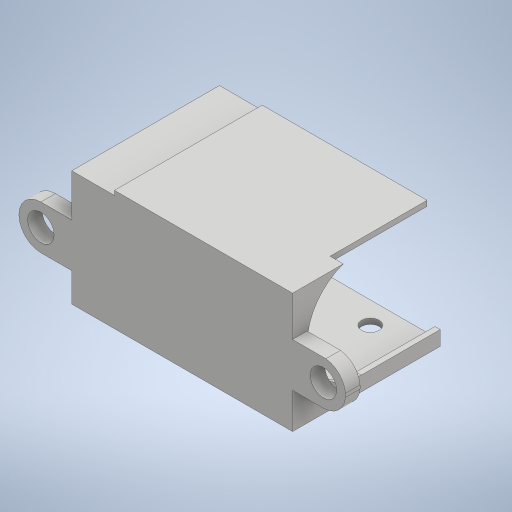
# Autodesk Inventor part: MotorMount
Saved by Autodesk Inventor 2023 (Build 270158000, 158)
## iProperties
Created: 2019-11-11
Part Number: MotorMount
Material: Generic
Document SubType Name: Modeling
Designer: neera
Density: 1 g/cm^3
Appearance: Default
Author: neera
Autodesk Inventor part; units mm, degrees
ref_plane "YZ Plane" through (0, 0, 0) normal (1, 0, 0) x (0, 1, 0)
ref_plane "XZ Plane" through (0, 0, 0) normal (0, 1, 0) x (-1, 0, 0)
ref_plane "XY Plane" through (0, 0, 0) normal (0, 0, 1) x (1, 0, 0)
sketch "Sketch1" plane through (0, 0, 0) normal (0, 1, 0) x (-1, 0, 0)
  line L0 (17.1623, 10.1297) -> (-30.5377, 10.1297)
  line L1 (-30.5377, 34.9297) -> (7.4623, 34.9297)
  line L2 (7.4623, 34.9297) -> (7.4623, 33.9297)
  line L3 (7.4623, 33.9297) -> (17.1623, 33.9297)
  line L4 (17.1623, 33.9297) -> (17.1623, 10.1297)
  line L5 (-31.7377, 8.9297) -> (18.3623, 8.9297)
  line L6 (18.3623, 8.9297) -> (18.3623, 35.1297)
  line L7 (18.3623, 35.1297) -> (8.6623, 35.1297)
  line L8 (8.6623, 35.1297) -> (8.6623, 36.1297)
  line L9 (8.6623, 36.1297) -> (-31.7377, 36.1297)
  line L10 (-30.5377, 10.1297) -> (-30.5377, 34.9297)
  line L11 (-31.7377, 8.9297) -> (-31.7377, 36.1297)
  point P0 (0, 0)
  dimension "d0" = 47.7
  dimension "d1" = 23.8
  dimension "d2" = 9.7
  dimension "d3" = 1
  dimension "d4" = 1.2
  dimension "d5" = 1.2
  dimension "d6" = 1.2
  dimension "d7" = 1.2
  dimension "d8" = 1.2
  dimension "d19" = 1.2
  constraints: 24 end point, 8 perpendicular, 2 horizontal
  measures "d0" distance of L0.start L0.end
  measures "d1" distance of L3.end L0.start
  measures "d2" distance of L2.end L3.end
  measures "d3" distance of L1.end L2.end
  measures "d4" distance between parallel lines of L0 L5
  measures "d5" distance between parallel lines of L6 L4
  measures "d6" distance between parallel lines of L3 L7
  measures "d7" distance between parallel lines of L2 L8
  measures "d8" distance between parallel lines of L1 L9
  measures "d19" distance between parallel lines of L10 L11
extrude "Extrusion3" add sketch "Sketch1" along normal blind 33.5
sketch "Sketch3" plane through (0, 0, 0) normal (0, -1, 0) x (1, 0, 0)
  line L0 (30.5377, 34.9297) -> (-7.4623, 34.9297) projected
  line L1 (30.5377, 34.9297) -> (30.5377, 10.1297) projected
  line L2 (30.5377, 34.9297) -> (30.5377, 10.1297)
  line L3 (-17.1623, 10.1297) -> (30.5377, 10.1297) projected
  line L4 (30.5377, 10.1297) -> (-17.1623, 10.1297)
  line L5 (-17.1623, 33.9297) -> (-17.1623, 10.1297) projected
  line L6 (-17.1623, 10.1297) -> (-17.1623, 33.9297)
  line L7 (-7.4623, 33.9297) -> (-7.4623, 34.9297) projected
  line L8 (-17.1623, 33.9297) -> (-7.4623, 33.9297)
  line L9 (-7.4623, 33.9297) -> (-7.4623, 34.9297)
  line L10 (-7.4623, 34.9297) -> (30.5377, 34.9297)
  point P0 (0, 0)
  constraints: 12 end point, 4 perpendicular, 2 collinear
extrude "Extrusion4" add sketch "Sketch3" against normal blind 1.2
sketch "Sketch4" plane through (31.7377, 0, 8.9297) normal (0, 0, -1) x (-1, 0, 0)
  arc A0 (29.9, 16.8) -> (38.3, 16.8) centre (34.1, 16.8) ccw
  line L0 (50.1, 0) -> (50.1, 33.5) projected
  line L1 (0, 0) -> (50.1, 0) projected
  line L2 (29.9, 16.8) -> (29.9, 33.5)
  line L3 (29.9, 33.5) -> (38.3, 33.5)
  line L4 (0, 33.5) -> (50.1, 33.5) projected
  line L5 (38.3, 33.5) -> (38.3, 16.8)
  circle A1 centre (43.65, 28.5) radius 2
  circle A2 centre (43.65, 8.5) radius 2
  circle A3 centre (10.85, 8.5) radius 2
  circle A4 centre (10.85, 28.5) radius 2
  point P0 (31.7377, 0)
  dimension "d24" = 16
  dimension "d25" = 16.8
  dimension "d26" = 4.2
  dimension "d27" = 4
  dimension "d28" = 6.45
  dimension "d29" = 5
  dimension "d30" = 4
  dimension "d31" = 6.45
  dimension "d32" = 20
  dimension "d33" = 4
  dimension "d34" = 4
  dimension "d35" = 32.8
  dimension "d36" = 20
  dimension "d37" = 5
  dimension "d38" = 0
  constraints: 6 end point, 5 centre point, 2 point on circle, 2 tangent, 2 vertical, 1 point on line
  measures "d24" distance from line of L0 A0.centre
  measures "d25" distance from line of L1 A0.centre
  measures "d26" radius of A0
  measures "d27" diameter of A1
  measures "d28" distance from line of L0 A1.centre
  measures "d29" distance from line of L4 A1.centre
  measures "d30" diameter of A2
  measures "d31" distance from line of L0 A2.centre
  measures "d32" distance of A1.centre A2.centre
  measures "d33" diameter of A3
  measures "d34" diameter of A4
  measures "d35" distance of A2.centre A3.centre
  measures "d36" distance of A3.centre A4.centre
  measures "d37" distance from line of A4.centre L4
  measures "d38" horizontal distance of A3.centre A4.centre
extrude "Extrusion5" cut sketch "Sketch4" against normal blind 5
sketch "Sketch5" plane through (31.7377, 0, 36.1297) normal (1, 0, 0) x (0, 0, -1)
  arc A0 (-0.7, 15.6) -> (23.9, 15.6) centre (11.6, 15.6) ccw
  line L0 (0, 0) -> (27.2, 0) projected
  line L1 (27.2, 0) -> (27.2, 33.5) projected
  line L2 (23.9, 15.6) -> (23.9, 33.5)
  line L3 (27.2, 33.5) -> (1, 33.5) projected
  line L4 (1, 33.5) -> (0, 33.5) projected
  line L5 (-0.7, 15.6) -> (18, 15.6) construction
  line L6 (0.1, 33.5) -> (23.9, 33.5)
  line L7 (-0.7, 15.6) -> (0, 15.6)
  line L8 (0, 0) -> (0, 33.5) projected
  line L9 (0, 15.6) -> (0, 33.5)
  line L10 (0, 33.5) -> (0.1, 33.5)
  point P0 (36.1297, 0)
  dimension "d41" = 24.6
  dimension "d42" = 15.6
  dimension "d43" = 15.6
  constraints: 12 end point, 2 collinear, 2 horizontal, 2 point on circle, 2 point on line, 1 centre point, 1 perpendicular, 1 vertical
  measures "d41" diameter of A0
  measures "d42" distance from line of L0 A0.centre
  measures "d43" distance from line of L1 A0.centre
extrude "Extrusion6" cut sketch "Sketch5" against normal blind 3 contours L7 L8 A0 | L8 L4 L3 L2 A0
sketch "Sketch6" plane through (0, 0, 0) normal (0, -1, 0) x (1, 0, 0)
  line L0 (39.3039, 27.0297) -> (31.7377, 27.0297)
  line L1 (31.7377, 27.0297) -> (31.7377, 17.0297)
  line L2 (31.7377, 17.0297) -> (38.7377, 17.0297)
  line L3 (43.7377, 21.6451) -> (43.7377, 22.4464)
  line L4 (31.7377, 36.1297) -> (31.7377, 8.9297) projected
  line L5 (31.7377, 8.9297) -> (-18.3623, 8.9297) projected
  arc A0 (38.7377, 17.0297) -> (39.3039, 27.0297) centre (38.7377, 22.0458) ccw
  line L6 (-18.3623, 8.9297) -> (-18.3623, 35.1297) projected
  line L7 (-18.3623, 25.5012) -> (-25.3623, 25.5012)
  line L8 (-30.3623, 15.5012) -> (-18.3623, 15.5012)
  line L9 (-18.3623, 15.5012) -> (-18.3623, 25.5012)
  arc A1 (-25.3623, 25.5012) -> (-25.3623, 15.5012) centre (-25.3623, 20.5012) ccw
  circle A2 centre (-25.3623, 20.5012) radius 3
  circle A3 centre (38.7377, 22.0458) radius 3
  point P0 (0, 0)
  dimension "d48" = 10
  dimension "d49" = 0
  dimension "d50" = 8.1
  dimension "d51" = 5
  dimension "d52" = 7
  dimension "d53" = 12
  dimension "d55" = 7
  dimension "d56" = 6
  dimension "d57" = 6
  constraints: 14 end point, 6 point on circle, 4 centre point, 3 parallel, 2 coincident, 2 horizontal, 2 point on line, 2 tangent, 1 perpendicular
  measures "d48" distance of L1.end L0.end
  measures "d49" distance between parallel lines of L4 L1
  measures "d50" distance between parallel lines of L5 L2
  measures "d51" distance from line of A0.centre L3
  measures "d52" distance from line of L4 A0.centre
  measures "d53" distance of L8.end L8.start
  measures "d55" distance from line of L6 A1.centre
  measures "d56" diameter of A2
  measures "d57" diameter of A3
extrude "Extrusion7" add sketch "Sketch6" against normal blind 3.3 contours A0 L3 L2 L1 L0 | L8 A1 L7 L6
body "Solid2"
